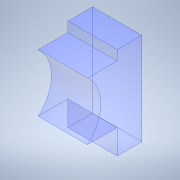
# Autodesk Inventor part: shank_2
Saved by Autodesk Inventor 2020.2 (Build 242310000, 310)
## iProperties
Created: 2021-01-30
Part Number: shank_2
Material: Generic
Document SubType Name: Modeling
Designer: DELL
Density: 1 g/cm^3
Appearance: Clear - Blue
Author: DELL
Autodesk Inventor part; units mm, degrees
ref_plane "Work Plane7" through (0, -46.2947, -99.445) normal (0, -0.9997, 0.0235) x (0, -0.0235, -0.9997)
ref_plane "Work Plane8" through (0, 70.92, -98.723) normal (0, -0.9994, -0.036) x (0, 0.036, -0.9994)
ref_plane "Work Plane9" through (-30, 0, 0) normal (1, 0, 0) x (0, 1, 0)
sketch "Sketch20" plane through (0, 0, 0) normal (1, 0, 0) x (0, 1, 0)
  line L0 (-87.4, 0) -> (69.4, 0) projected
  line L1 (0, -124.4) -> (0, 74.4) construction
  circle A0 centre (0, 0) radius 40
  circle A1 centre (0, 0) radius 46
  line L2 (35, -29.8496) -> (35, -66)
  line L3 (-35, -66) -> (-35, -29.8496)
  line L4 (47, -66) -> (-65, -66)
  line L5 (47, -66) -> (47, -96)
  line L6 (47, -96) -> (-65, -96)
  line L7 (-65, -96) -> (-65, -66)
  point P0 (0, -66)
  dimension "d254" = 92
  dimension "d255" = 80
  dimension "d256" = 70
  dimension "d261" = 90
  dimension "d262" = 30
  dimension "d263" = 47
  dimension "d264" = 65
  dimension "d265" = 96
  dimension "d268" = 30
  dimension "d269" = 12
  dimension "d273" = 36.1504
  constraints: 12 end point, 4 point on line, 2 centre point, 2 coincident, 2 parallel, 2 point on circle, 1 perpendicular, 1 vertical, 1 other
  measures "d254" diameter of A1
  measures "d255" diameter of A0
  measures "d256" distance between parallel lines of L2 L3
  measures "d261" angle of L1 L4
  measures "d262" distance of L4.start L5.end
  measures "d263" distance of L4.start point (0, -66)
  measures "d264" distance of L4.end point (0, -66)
  measures "d265" distance from line of L6 point (0, 0)
  measures "d268" distance of L4.end L3.start
  measures "d269" distance of L4.start L2.end
  measures "d273" distance of L2.start L2.end
extrude "Extrusion18" add sketch "Sketch20" along normal mid plane 60 contours L2 L4 L3 A1 | L4 L5 L6 L7
sketch "Sketch21" plane through (-30, 47, -66) normal (0, 1, 0) x (1, 0, 0)
  line L0 (0, 0) -> (60, 0) projected
  line L1 (60, 30) -> (60, 0) projected
  line L2 (0, 30) -> (60, 30) projected
  line L3 (0, 0) -> (0, 30) projected
  line L4 (60, 30) -> (60, 0) projected
  line L5 (0, 0) -> (0, 30) projected
  arc A0 (60, 1029.0992) -> (0, 1029.0992) centre (30, 530) ccw
  line L6 (0, 30) -> (60, 30) projected
  point P0 (30, 30)
  point P1 (60, 29.0992)
  point P2 (0, 29.0992)
  dimension "d270" = 500
  constraints: 2 point on circle, 2 point on line, 1 centre point, 1 horizontal alignment, 1 tangent
  measures "d270" radius of A0
sketch3d "3D Sketch1"
  constraints: 14 end point, 12 point on circle, 4 centre point, 4 line through centre, 3 point on line, 2 coincident, 2 perpendicular, 1 tangent, 1 vertical, 3 other
body "Solid1"
body "Solid8"
body "Solid9"
